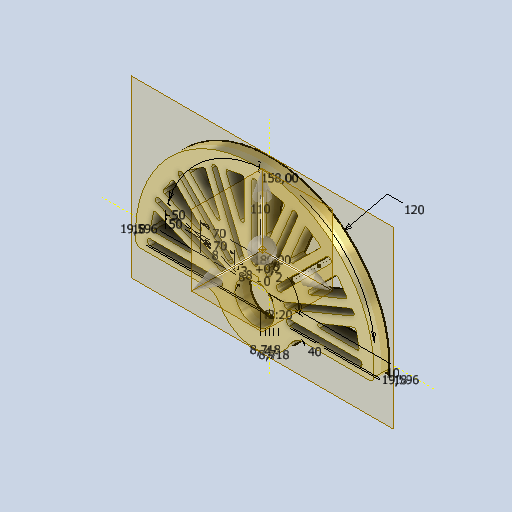
# Autodesk Inventor part: Capstonradialdisc
Saved by Autodesk Inventor 2022 (Build 260153000, 153)
## iProperties
Created: 2022-03-11
Part Number: Capstonradialdisc
Material: Generisch
Document SubType Name: Modeling
Designer: 123St
Density: 1 g/cm^3
Appearance: Gold - Metall
Mass: 270.626 g
Surface Area: 814.649 cm^2
Volume: 270.626 cm^3
CapstonDisc_Thickness: 15,000 mm
CapstonBig_Radius: 120,000 mm
Author: 123St
Autodesk Inventor part; units mm, degrees
ref_plane "YZ Plane" through (0, 0, 0) normal (1, 0, 0) x (0, 1, 0)
ref_plane "XZ Plane" through (0, 0, 0) normal (0, 1, 0) x (-1, 0, 0)
ref_plane "XY Plane" through (0, 0, 0) normal (0, 0, 1) x (1, 0, 0)
sketch "Skizze1" plane through (0, 0, 0) normal (0, 0, 1) x (1, 0, 0)
  line L0 (-4, 24) -> (4, 24)
  line L1 (4, 24) -> (4, 19.5959)
  line L2 (-4, 19.5959) -> (-4, 24)
  line L3 (-4, 24) -> (4, 19.5959) construction
  line L4 (4, 24) -> (-4, 19.5959) construction
  line L5 (0, 152) -> (0, -72) construction
  line L6 (-168, 0) -> (168, 0) construction
  line L7 (-35, 0) -> (-105, 0) construction
  line L8 (-35, -3) -> (-105, -3)
  line L9 (-105, 3) -> (-35, 3)
  arc A0 (-35, -3) -> (-35, 3) centre (-35, 0) ccw
  arc A1 (-105, 3) -> (-105, -3) centre (-105, 0) ccw
  arc A2 (-38.7298, -10) -> (38.7298, -10) centre (0, 0) ccw
  line L10 (-38.7298, -10) -> (-119.5826, -10)
  line L11 (38.7298, -10) -> (119.5826, -10)
  arc A3 (119.5826, -10) -> (-119.5826, -10) centre (0, 0) ccw
  arc A4 (-33.4838, 10.6223) -> (-31.1877, 16.1656) centre (-32.3358, 13.3939) ccw
  line L12 (-95.8593, 42.9534) -> (-31.1877, 16.1656)
  line L13 (-32.3358, 13.3939) -> (-97.0074, 40.1818) construction
  arc A5 (-95.8593, 42.9534) -> (-98.1554, 37.4101) centre (-97.0074, 40.1818) ccw
  line L14 (-33.4838, 10.6223) -> (-98.1554, 37.4101)
  arc A6 (-26.8701, 22.6274) -> (-22.6274, 26.8701) centre (-24.7487, 24.7487) ccw
  line L15 (-72.1249, 76.3675) -> (-22.6274, 26.8701)
  line L16 (-24.7487, 24.7487) -> (-74.2462, 74.2462) construction
  arc A7 (-72.1249, 76.3675) -> (-76.3675, 72.1249) centre (-74.2462, 74.2462) ccw
  line L17 (-26.8701, 22.6274) -> (-76.3675, 72.1249)
  arc A8 (-16.1656, 31.1877) -> (-10.6223, 33.4838) centre (-13.3939, 32.3358) ccw
  line L18 (-37.4101, 98.1554) -> (-10.6223, 33.4838)
  line L19 (-13.3939, 32.3358) -> (-40.1818, 97.0074) construction
  arc A9 (-37.4101, 98.1554) -> (-42.9534, 95.8593) centre (-40.1818, 97.0074) ccw
  line L20 (-16.1656, 31.1877) -> (-42.9534, 95.8593)
  arc A10 (-3, 35) -> (3, 35) centre (0, 35) ccw
  line L21 (3, 105) -> (3, 35)
  line L22 (0, 35) -> (0, 105) construction
  arc A11 (3, 105) -> (-3, 105) centre (0, 105) ccw
  line L23 (-3, 35) -> (-3, 105)
  arc A12 (10.6223, 33.4838) -> (16.1656, 31.1877) centre (13.3939, 32.3358) ccw
  line L24 (42.9534, 95.8593) -> (16.1656, 31.1877)
  line L25 (13.3939, 32.3358) -> (40.1818, 97.0074) construction
  arc A13 (42.9534, 95.8593) -> (37.4101, 98.1554) centre (40.1818, 97.0074) ccw
  line L26 (10.6223, 33.4838) -> (37.4101, 98.1554)
  arc A14 (22.6274, 26.8701) -> (26.8701, 22.6274) centre (24.7487, 24.7487) ccw
  line L27 (76.3675, 72.1249) -> (26.8701, 22.6274)
  line L28 (24.7487, 24.7487) -> (74.2462, 74.2462) construction
  arc A15 (76.3675, 72.1249) -> (72.1249, 76.3675) centre (74.2462, 74.2462) ccw
  line L29 (22.6274, 26.8701) -> (72.1249, 76.3675)
  arc A16 (31.1877, 16.1656) -> (33.4838, 10.6223) centre (32.3358, 13.3939) ccw
  line L30 (98.1554, 37.4101) -> (33.4838, 10.6223)
  line L31 (32.3358, 13.3939) -> (97.0074, 40.1818) construction
  arc A17 (98.1554, 37.4101) -> (95.8593, 42.9534) centre (97.0074, 40.1818) ccw
  line L32 (31.1877, 16.1656) -> (95.8593, 42.9534)
  arc A18 (35, 3) -> (35, -3) centre (35, 0) ccw
  line L33 (105, -3) -> (35, -3)
  line L34 (35, 0) -> (105, 0) construction
  arc A19 (105, -3) -> (105, 3) centre (105, 0) ccw
  line L35 (35, 3) -> (105, 3)
  line L36 (-55.3007, 11) -> (-101.4947, 30.1342)
  line L37 (-101.4947, 30.1342) -> (-105.3007, 11)
  line L38 (-105.3007, 11) -> (-55.3007, 11)
  line L39 (-82.1538, 66.7832) -> (-93.0127, 50.5755)
  line L40 (-46.8426, 31.3838) -> (-82.1538, 66.7832)
  line L41 (-93.0127, 50.5755) -> (-46.8426, 31.3838)
  line L42 (-50.2273, 93.2012) -> (-66.4754, 82.403)
  line L43 (-31.2084, 46.9597) -> (-50.2273, 93.2012)
  line L44 (-66.4754, 82.403) -> (-31.2084, 46.9597)
  line L45 (-10.6061, 105.3411) -> (-29.7544, 101.6067)
  line L46 (-10.7931, 55.3415) -> (-10.6061, 105.3411)
  line L47 (-29.7544, 101.6067) -> (-10.7931, 55.3415)
  line L48 (30.6399, 101.3432) -> (11.525, 105.2446)
  line L49 (11.2756, 55.2452) -> (30.6399, 101.3432)
  line L50 (11.525, 105.2446) -> (11.2756, 55.2452)
  line L51 (67.192, 81.8198) -> (51.0387, 92.7593)
  line L52 (31.617, 46.6855) -> (67.192, 81.8198)
  line L53 (51.0387, 92.7593) -> (31.617, 46.6855)
  line L54 (93.4505, 49.7619) -> (82.7335, 66.0637)
  line L55 (47.1147, 30.9738) -> (93.4505, 49.7619)
  line L56 (82.7335, 66.0637) -> (47.1147, 30.9738)
  line L57 (105.3927, 10.0807) -> (101.7538, 29.2473)
  line L58 (55.3946, 10.517) -> (105.3927, 10.0807)
  line L59 (101.7538, 29.2473) -> (55.3946, 10.517)
  circle A20 centre (0, 0) radius 20
  line L60 (0, 20) -> (4, 20) construction
  line L61 (-4, -24) -> (4, -24)
  line L62 (4, -24) -> (4, -19.5959)
  line L63 (-4, -19.5959) -> (-4, -24)
  line L64 (-4, -24) -> (4, -19.5959) construction
  line L65 (4, -24) -> (-4, -19.5959) construction
  line L66 (0, -20) -> (4, -20) construction
  arc A21 (-4, 19.5959) -> (-4, -19.5959) centre (0, 0) ccw
  arc A22 (4, -19.5959) -> (4, 19.5959) centre (0, 0) ccw
  line L67 (-8.7178, -18) -> (8.7178, -18)
  line L68 (-8.7178, 18) -> (8.7178, 18)
  point P0 (0, 21.798)
  point P1 (-70, 0)
  point P2 (-64.6716, 26.7878)
  point P3 (-49.4975, 49.4975)
  point P4 (-26.7878, 64.6716)
  point P5 (0, 70)
  point P6 (26.7878, 64.6716)
  point P7 (49.4975, 49.4975)
  point P8 (64.6716, 26.7878)
  point P9 (70, 0)
  point P10 (0, -21.798)
  point P11 (4, -19.5959)
  point P12 (-4, -19.5959)
  point P13 (0, 110)
  point P14 (0, 32)
  point P15 (-8.7178, 18)
  point P16 (8.7178, 18)
  dimension "d2" = 8
  dimension "d7" = 70
  dimension "d8" = 3
  dimension "d9" = 70
  dimension "d12" = 180
  dimension "CapstonBig_Radius" = 120
  dimension "d19" = 40
  dimension "d21" = 8
  dimension "d22" = 8
  dimension "d23" = 50
  dimension "d24" = 50
  dimension "d27" = 158
  dimension "d43" = 20
  dimension "d44" = 10
  dimension "d45" = 110
  dimension "d53" = 2
  dimension "d54" = 8
  dimension "d55" = 18
  dimension "d56" = 8.7178
  dimension "d57" = 19.5959
  dimension "d58" = 4
  dimension "d59" = 19.5959
  dimension "d60" = 4
  dimension "d61" = 18
  dimension "d62" = 8.7178
  dimension "d63" = 2
  constraints: 152 end point, 51 point on circle, 23 centre point, 8 point on line, 7 symmetric about line, 6 coincident, 6 tangent, 5 midpoint, 5 parallel, 4 horizontal, 2 perpendicular, 147 other
  measures "d2" distance of L0.start L0.end
  measures "d7" distance of L9.start L9.end
  measures "d8" radius of A0
  measures "d9" distance of point (0, 0) point (-70, 0)
  measures "CapstonBig_Radius" radius of A3
  measures "d19" radius of A2
  measures "d21" distance between parallel lines of L9 L38
  measures "d22" distance between parallel lines of L14 L36
  measures "d23" distance of L37.end L36.start
  measures "d24" distance of L36.start L36.end
  measures "d43" radius of A22
  measures "d44" distance between parallel lines of L11 L6
  measures "d45" distance of point (0, 0) point (0, 110)
  measures "d53" distance from line of L67 L66.start
  measures "d54" distance from line of point (0, 32) L0
  measures "d55" distance from line of point (8.718, -18) L6
  measures "d56" distance from line of point (8.718, -18) L5
  measures "d57" distance from line of point (4, -19.596) L6
  measures "d58" distance from line of point (4, -19.596) L5
  measures "d59" distance from line of point (-4, -19.596) L6
  measures "d60" distance from line of point (-4, -19.596) L5
  measures "d61" distance from line of point (-8.718, -18) L6
  measures "d62" distance from line of point (-8.718, -18) L5
  measures "d63" distance from line of L68 L60.start
extrude "Extrusion1" add sketch "Skizze1" along normal blind 15 contours A20 L62 L61 L63 | L10 A3 L11 A2
extrude "Extrusion3" add sketch "Skizze1" along normal blind 15 separate body contours L0 L1 A20 L2 | A20 L68
fillet "Rundung1" radius 15 2 edges at (-38.7298, -10, 7.5) (38.7298, -10, 7.5)
fillet "Rundung2" radius 5 2 edges at (119.5826, -10, 7.5) (-119.5826, -10, 7.5)
sketch "Skizze2" plane through (48.9898, -10, 0) normal (0, -1, 0) x (1, 0, 0)
  circle A0 centre (62.8967, 2.5) radius 1
  line L0 (0, 0) -> (65.9015, 0) projected
  circle A1 centre (-160.8763, 12.5) radius 1
  line L1 (-163.881, 15) -> (-97.9796, 15) projected
  line L2 (-168.8763, 15) -> (-168.8763, 0) projected
  line L3 (70.8967, 0) -> (70.8967, 15) projected
  point P0 (-48.9898, 0)
  dimension "d29" = 2.5
  dimension "d30" = 2
  dimension "d31" = 2.5
  dimension "d32" = 2
  dimension "d33" = 8
  dimension "d34" = 8
  constraints: 2 centre point
  measures "d29" distance from line of L0 A0.centre
  measures "d30" diameter of A0
  measures "d31" distance from line of L1 A1.centre
  measures "d32" diameter of A1
  measures "d33" distance from line of L2 A1.centre
  measures "d34" distance from line of L3 A0.centre
extrude "Extrusion2" cut sketch "Skizze2" against normal blind 15 bodies 1
fillet "Rundung3" radius 2 24 edges at (-101.4947, 30.1342, 7.5) (-105.3007, 11, 7.5) (-93.0127, 50.5755, 7.5) (-66.4754, 82.403, 7.5) (-10.6061, 105.3411, 7.5) (-50.2273, 93.2012, 7.5) (-82.1538, 66.7832, 7.5) (-29.7544, 101.6067, 7.5) (30.6399, 101.3432, 7.5) (11.525, 105.2446, 7.5) (67.192, 81.8198, 7.5) (51.0387, 92.7593, 7.5) (93.4505, 49.7619, 7.5) (82.7335, 66.0637, 7.5) (101.7538, 29.2473, 7.5) (105.3927, 10.0807, 7.5) (-55.3007, 11, 7.5) (-46.8426, 31.3838, 7.5) (-31.2084, 46.9597, 7.5) (-10.7931, 55.3415, 7.5) (11.2756, 55.2452, 7.5) (31.617, 46.6855, 7.5) (47.1147, 30.9738, 7.5) (55.3946, 10.517, 7.5)
ref_plane "Arbeitsebene1" through (0, 0, 7.5) normal (0, 0, 1) x (1, 0, 0)
equation "\"d43\" = Shaft_CapstonPart_Dia"
equation "\"Shaft_CapstonPart_Dia\" = 20"
